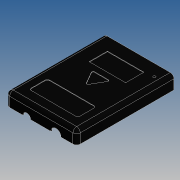
# Autodesk Inventor part: P127
Saved by Autodesk Inventor 2019 (Build 230136000, 136)
## iProperties
Created: 2017-01-31
Part Number: P127
Material: ABS Plastic
Document SubType Name: Modeling
Designer: serge.amoos
Density: 1.06 g/cm^3
Appearance: Smooth - Black
Description: Couvercle compartiment  laser
Author: serge.amoos
Autodesk Inventor part; units mm, degrees
ref_plane "YZ Plane" through (0, 0, 0) normal (1, 0, 0) x (0, 1, 0)
ref_plane "XZ Plane" through (0, 0, 0) normal (0, 1, 0) x (-1, 0, 0)
ref_plane "XY Plane" through (0, 0, 0) normal (0, 0, 1) x (1, 0, 0)
sketch "Sketch1" plane through (0, 0, 0) normal (0, 0, 1) x (1, 0, 0)
  line L0 (-34.8, 0) -> (5.8, 0) construction
  line L1 (0, -8) -> (0, 48) construction
  line L2 (0, 0) -> (-29, 0)
  line L3 (-29, 0) -> (-29, 40)
  line L4 (-29, 40) -> (0, 40)
  line L5 (0, 40) -> (0, 0)
  dimension "d0" = 29
  dimension "d1" = 40
  constraints: 8 end point, 2 parallel, 1 horizontal, 1 perpendicular
  measures "d0" distance of L3.end L4.end
  measures "d1" distance of L2.end L3.end
extrude "Extrusion1" add sketch "Sketch1" along normal blind 11
shell "Shell1" thickness 2 removed faces 3 at (-9.6667, 13.3333, 0) at (-9.6667, 0, 3.6667) at (0, 26.6667, 3.6667)
sketch "Sketch2" plane through (0, 0, 0) normal (0, 0, -1) x (-1, 0, 0)
  line L0 (34.8, 0) -> (-5.8, 0) construction
  line L1 (0, -8) -> (0, 48) construction
  line L2 (27, 38) -> (27, 0) projected
  line L3 (0, 38) -> (27, 38) projected
  line L4 (28, 0) -> (28, 39)
  line L5 (28, 39) -> (0, 39)
  line L6 (28, 0) -> (27, 0)
  line L7 (0, 38) -> (0, 39)
  point P0 (0, 0)
  dimension "d7" = 1
  dimension "d18" = 1
  constraints: 8 end point, 2 horizontal, 1 collinear
  measures "d7" distance between parallel lines of L2 L4
  measures "d18" distance between parallel lines of L3 L5
extrude "Extrusion2" cut sketch "Sketch2" against normal blind 2
sketch "Sketch3" plane through (0, 0, 0) normal (0, 0, -1) x (-1, 0, 0)
  line L0 (28, 39) -> (28, 0) construction
  line L1 (0, 39) -> (28, 39) construction
  line L2 (34.8, 0) -> (-5.8, 0) construction
  line L3 (0, -8) -> (0, 48) construction
  line L4 (28, 20) -> (27.8, 20)
  line L5 (27.8, 20) -> (27.8, 30)
  line L6 (27.8, 30) -> (28, 30)
  line L7 (28, 30) -> (28, 20)
  line L8 (5, 39) -> (0, 39)
  line L9 (0, 39) -> (0, 38.8)
  line L10 (0, 38.8) -> (5, 38.8)
  line L11 (5, 38.8) -> (5, 39)
  point P0 (0, 0)
  point P1 (28, 37)
  point P2 (26, 39)
  dimension "d10" = 10
  dimension "d11" = 20
  dimension "d12" = 0.2
  dimension "d13" = 5
  dimension "d14" = 0.2
  constraints: 16 end point, 4 parallel, 3 point on line, 2 horizontal, 2 perpendicular
  measures "d10" distance of L4.end L5.end
  measures "d11" distance from line of L4.end L2
  measures "d12" distance between parallel lines of L0 L5
  measures "d13" distance of L9.end L10.end
  measures "d14" distance between parallel lines of L1 L10
extrude "Extrusion3" add sketch "Sketch3" against normal blind 0.8
fillet "Fillet3" radius 0.2 2 edges at (-27.8, 25, 0.8) (-2.5, 38.8, 0.8)
mirror "Mirror1" about plane through (-29, 0, 0) normal (0, -1, 0)
mirror "Mirror2" about plane through (0, 0, 0) normal (1, 0, 0)
fillet "Fillet4" radius 1 4 edges at (27, -38, 5.5) (-27, -38, 5.5) (-27, 38, 5.5) (27, 38, 5.5)
fillet "Fillet5" radius 3 2 edges at (-29, -40, 5.5) (29, -40, 5.5)
fillet "Fillet6" radius 3 5 edges at (-28.1213, -39.1213, 11) (0, -40, 11) (28.1213, -39.1213, 11) (29, 1.5, 11) (-29, 1.5, 11)
sketch "Sketch4" plane through (-26, -40, 0) normal (0, -1, 0) x (1, 0, 0)
  line L0 (-14.6, 0) -> (66.6, 0) construction
  line L1 (26, -2.2) -> (26, 13.2) construction
  arc A0 (42.2, 0) -> (33.8, 0) centre (38, 0) ccw
  arc A1 (17.2, 0) -> (10.8, 0) centre (14, 0) ccw
  line L2 (10.8, 0) -> (17.2, 0)
  line L3 (33.8, 0) -> (42.2, 0)
  point P0 (26, 0)
  dimension "d22" = 12
  dimension "d23" = 12
  dimension "d24" = 4.2
  dimension "d25" = 3.2
  constraints: 4 end point, 4 point on circle, 4 point on line, 2 centre point, 2 collinear
  measures "d22" distance from line of A0.centre L1
  measures "d23" distance from line of L1 A1.centre
  measures "d24" radius of A0
  measures "d25" radius of A1
extrude "Extrusion4" cut sketch "Sketch4" against normal blind 10
sketch "Sketch5" plane through (-26, 38, 9) normal (0, -1, 0) x (1, 0, 0)
  line L0 (54, -7) -> (-2, -7) projected
  line L1 (-2, -9) -> (-2, -7) projected
  line L2 (21, -9) -> (-2, -9) projected
  arc A0 (5, -9) -> (1, -9) centre (3, -9) ccw
  line L3 (1, -9) -> (5, -9)
  point P0 (26, -9)
  dimension "d32" = 2
  dimension "d33" = 3
  constraints: 2 end point, 2 point on circle, 2 point on line, 1 centre point, 1 collinear
  measures "d32" radius of A0
  measures "d33" distance of L1.start L3.start
extrude "Extrusion6" cut sketch "Sketch5" against normal through all contours A0 L2
fillet "Fillet7" radius 2 4 edges at (-28, 39, 1) (28, 39, 1) (-28, -39, 1) (28, -39, 1)
sketch "Sketch6" plane through (0, 0, 0) normal (0, 0, -1) x (-1, 0, 0)
  line L0 (-29, -37) -> (-29, 40) projected
  line L1 (21, 40) -> (-29, 40) projected
  point P0 (0, 0)
  point P1 (-22.5, 30.4)
  dimension "d37" = 6.5
  dimension "d38" = 9.6
  measures "d37" distance from line of point (-22.5, 30.4) L0
  measures "d38" distance from line of L1 point (-22.5, 30.4)
hole "Hole1" at (22.5, 30.4, 0) direction (0, 0, 1) diameter 2 end through all
sketch "Sketch7" plane through (0, 0, 11) normal (0, 0, 1) x (1, 0, 0)
  line L0 (-40.6, 0) -> (40.6, 0) construction
  line L1 (0, -56) -> (0, 56) construction
  line L2 (20, -30) -> (-20, -30)
  line L3 (-20, -30) -> (-20, -15)
  line L4 (-20, -15) -> (20, -15)
  line L5 (20, -15) -> (20, -30)
  line L6 (-26, -40) -> (26, -40) construction
  line L7 (0, -3.6603) -> (-7.5, 9.3301)
  line L8 (-7.5, 9.3301) -> (7.5, 9.3301)
  line L9 (7.5, 9.3301) -> (0, -3.6603)
  line L10 (15, 14.3301) -> (-15, 14.3301)
  line L11 (-15, 14.3301) -> (-15, 29.3301)
  line L12 (-15, 29.3301) -> (15, 29.3301)
  line L13 (15, 29.3301) -> (15, 14.3301)
  point P0 (0, 0)
  point P1 (0, -30)
  point P2 (0, 5)
  point P3 (0, 14.3301)
  dimension "d46" = 40
  dimension "d47" = 15
  dimension "d48" = 10
  dimension "d49" = 15
  dimension "d51" = 5
  dimension "d52" = 30
  dimension "d53" = 15
  dimension "d54" = 5
  constraints: 22 end point, 4 parallel, 3 horizontal, 3 point on line, 2 midpoint, 2 perpendicular, 7 other
  measures "d46" distance of L2.start L2.end
  measures "d47" distance of L2.end L3.end
  measures "d48" distance between parallel lines of L2 L6
  measures "d49" distance of L7.start L7.end
  measures "d51" distance from line of point (0, 5) L0
  measures "d52" distance of L10.start L10.end
  measures "d53" distance of L10.end L11.end
  measures "d54" distance between parallel lines of L10 L8
extrude "Extrusion7" cut sketch "Sketch7" against normal blind 0.4
fillet "Fillet8" radius 2 4 edges at (20, -30, 10.8) (-20, -30, 10.8) (-20, -15, 10.8) (20, -15, 10.8)
fillet "Fillet9" radius 1 3 edges at (0, -3.6603, 10.8) (7.5, 9.3301, 10.8) (-7.5, 9.3301, 10.8)
equation "\"d23\" = d22"
body "Solid1"
